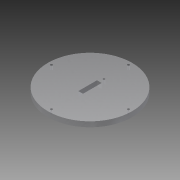
# Autodesk Inventor part: open1
Saved by Autodesk Inventor 2015 (Build 190159000, 159)
## iProperties
Created: 2015-02-17
Part Number: open1
Material: Plastic, Transparent
Document SubType Name: Modeling
Designer: Hanjie
Density: 1.188 g/cm^3
Appearance: Transparent - Clear
Author: Hanjie
Autodesk Inventor part; units mm, degrees
ref_plane "YZ Plane" through (0, 0, 0) normal (1, 0, 0) x (0, 1, 0)
ref_plane "XZ Plane" through (0, 0, 0) normal (0, 1, 0) x (-1, 0, 0)
ref_plane "XY Plane" through (0, 0, 0) normal (0, 0, 1) x (1, 0, 0)
sketch "Sketch1" plane through (0, 0, 0) normal (0, 1, 0) x (-1, 0, 0)
  circle A0 centre (0, 0) radius 45.72
  dimension "d0" = 91.44
  constraints: 1 centre point, 1 coincident
  measures "d0" diameter of A0
extrude "Extrusion1" add sketch "Sketch1" along normal blind 5.588
sketch "Sketch2" plane through (0, 5.588, 0) normal (0, 1, 0) x (1, 0, 0)
  circle A0 centre (0, 0) radius 38.1
  line L0 (0, 0) -> (-41.91, 0)
  line L1 (0, 0) -> (0, 41.91)
  line L2 (0, 0) -> (41.91, 0)
  line L3 (0, 0) -> (0, -41.91)
  circle A1 centre (-41.91, 0) radius 1.27
  circle A2 centre (0, -41.91) radius 1.27
  circle A3 centre (0, 41.91) radius 1.27
  circle A4 centre (41.91, 0) radius 1.27
  line L4 (0, 0) -> (0, -10.16)
  line L5 (0, -10.16) -> (-2.54, -10.16)
  line L6 (-2.54, -10.16) -> (2.54, -10.16)
  line L7 (2.54, -10.16) -> (2.54, 10.16)
  line L8 (2.54, 10.16) -> (-2.54, 10.16)
  line L9 (-2.54, 10.16) -> (-2.54, -10.16)
  line L10 (0, 0) -> (0, 15.24)
  circle A5 centre (0, 15.24) radius 1.016
  dimension "d3" = 76.2
  dimension "d4" = 41.91
  dimension "d5" = 41.91
  dimension "d6" = 41.91
  dimension "d7" = 41.91
  dimension "d8" = 2.54
  dimension "d9" = 2.54
  dimension "d10" = 2.54
  dimension "d11" = 2.54
  dimension "d12" = 10.16
  dimension "d13" = 2.54
  dimension "d14" = 5.08
  dimension "d15" = 20.32
  dimension "d16" = 15.24
  dimension "d17" = 2.032
  constraints: 22 end point, 6 centre point, 6 coincident, 3 horizontal, 3 perpendicular, 2 parallel, 2 point on line, 1 vertical
  measures "d3" diameter of A0
  measures "d4" distance of L0.start L0.end
  measures "d5" distance of L0.start L1.end
  measures "d6" distance of L0.start L2.end
  measures "d7" distance of L0.start L3.end
  measures "d8" diameter of A1
  measures "d9" diameter of A2
  measures "d10" diameter of A3
  measures "d11" diameter of A4
  measures "d12" distance of L0.start L4.end
  measures "d13" distance of L4.end L5.end
  measures "d14" distance of L8.end L7.end
  measures "d15" distance of L7.end L6.end
  measures "d16" distance of L0.start L10.end
  measures "d17" diameter of A5
extrude "Extrusion2" cut sketch "Sketch2" against normal blind 5.588 contours A2 | A1 | A3 | A4 | L7 L6 L3 L2 | L2 L1 L8 L7 | A5 L1 | L1 A5 | L5 L9 L0 L3 | L0 L9 L8 L1
body "Solid1"
